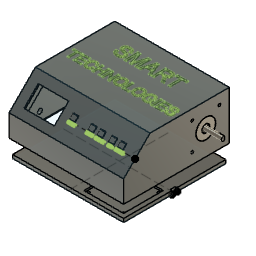
Stepper motor box v1 (Autodesk Fusion 360 design; units mm, degrees)
Autodesk Fusion 360 part; units mm, degrees
(part 1 of 3)
sketch "Sketch1" plane through (0, 0, 0) normal (0, 0, 1) x (1, 0, 0) in component "Stepper Motor"
  line L0 (21.15, -21.15) -> (-21.15, -21.15)
  line L1 (-21.15, -21.15) -> (-21.15, 21.15)
  line L2 (-21.15, 21.15) -> (21.15, 21.15)
  line L3 (21.15, 21.15) -> (21.15, -21.15)
  line L4 (21.15, -21.15) -> (-21.15, 21.15) construction
  line L5 (-21.15, -21.15) -> (21.15, 21.15) construction
  dimension "d2" = 42.3
  dimension "d3" = 42.3
  constraint horizontal L0
  constraint perpendicular L0 L1
  constraint parallel L0 L2
  constraint parallel L1 L3
  constraint coincident L4 origin
  constraint coincident L5 origin
  measures "d2" distance of L1.end L2.end
  measures "d3" distance of L0.end L1.end
extrude "Extrude1" add sketch "Sketch1" along normal blind 23 makes body 1 in component "Stepper Motor"
sketch "Sketch2" plane through (0, 0, 23) normal (0, 0, 1) x (-1, 0, 0) in component "Stepper Motor"
  line L0 (-21.15, -21.15) -> (21.15, -21.15)
  line L1 (21.15, -21.15) -> (21.15, 21.15)
  line L2 (21.15, 21.15) -> (-21.15, 21.15)
  line L3 (-21.15, 21.15) -> (-21.15, -21.15)
  circle A0 centre (0, 0) radius 11
  dimension "d6" = 22
  constraint coincident A0.centre origin
  measures "d6" diameter of A0
extrude "Extrude2" add sketch "Sketch2" along normal blind 2 contours A0 bodies 1 in component "Stepper Motor"
sketch "Sketch3" plane through (0, 0, 25) normal (0, 0, 1) x (-1, 0, 0) in component "Stepper Motor"
  circle A0 centre (0, 0) radius 11
  circle A1 centre (0, 0) radius 4.5
  dimension "d9" = 9
  constraint concentric A0 A1
  measures "d9" diameter of A1
extrude "Extrude3" cut sketch "Sketch3" against normal blind 2 contours A1 bodies 1 in component "Stepper Motor"
sketch "Sketch5" plane through (0, 0, 23) normal (0, 0, 1) x (-1, 0, 0) in component "Stepper Motor"
  circle A0 centre (0, 0) radius 4.5
  circle A1 centre (0, 0) radius 2.5
  dimension "d12" = 5
  constraint coincident A0.centre A1.centre
  measures "d12" diameter of A1
extrude "Extrude4" add sketch "Sketch5" along normal blind 22 contours A1 bodies 1 in component "Stepper Motor"
sketch "Sketch6" plane through (0, 0, 45) normal (0, 0, 1) x (-1, 0, 0) in component "Stepper Motor"
  circle A0 centre (0, 0) radius 2.5
  line L0 (2.1585, -1.2614) -> (-2.1585, -1.2614)
  dimension "d15" = 1.2614
  constraint coincident A0 L0.start
  constraint coincident A0 L0.end
  constraint horizontal L0
  measures "d15" distance of A0.centre L0
extrude "Extrude5" cut sketch "Sketch6" against normal blind 6 contours A0 L0 picked at (-0.5645, -1.4539) bodies 1 in component "Stepper Motor"
sketch "Sketch7" plane through (0, 0, 23) normal (0, 0, 1) x (-1, 0, 0) in component "Stepper Motor"
  circle A0 centre (0, 0) radius 11
  line L0 (-21.15, -21.15) -> (21.15, -21.15)
  line L1 (21.15, -21.15) -> (21.15, 21.15)
  line L2 (21.15, 21.15) -> (-21.15, 21.15)
  line L3 (-21.15, 21.15) -> (-21.15, -21.15)
  circle A1 centre (-15.5, -15.5) radius 1.5
  circle A2 centre (15.5, -15.5) radius 1.5
  circle A3 centre (-15.5, 15.5) radius 1.5
  circle A4 centre (15.5, 15.5) radius 1.5
  dimension "d18" = 3
  dimension "d19" = 3
  dimension "d20" = 3
  dimension "d21" = 3
  dimension "d27" = 5.65
  dimension "d28" = 5.65
  dimension "d29" = 5.65
  dimension "d30" = 5.65
  dimension "d32" = 5.65
  dimension "d33" = 5.65
  dimension "d34" = 5.65
  dimension "d35" = 5.65
  measures "d18" diameter of A1
  measures "d19" diameter of A2
  measures "d20" diameter of A3
  measures "d21" diameter of A4
  measures "d27" distance of L3 A3.centre
  measures "d28" distance of L2 A3.centre
  measures "d29" distance of L1 A2.centre
  measures "d30" distance of L0 A2.centre
  measures "d32" distance of L3 A1.centre
  measures "d33" distance of L0 A1.centre
  measures "d34" distance of L2 A4.centre
  measures "d35" distance of L1 A4.centre
extrude "Extrude6" cut sketch "Sketch7" against normal blind 4.5 contours A1 | A2 | A3 | A4 bodies 1 in component "Stepper Motor"
thread "Thread1" "ISO Metric profile 3.0 M3x0.5 6H" major diameter 3.086 minor diameter 2.529 pitch 0.5 angle 60 resizes the face on face at (14.0019, 15.5748, 20) on bodies 1 in component "Stepper Motor"
thread "Thread2" "ISO Metric profile 3.0 M3x0.5 6H" major diameter 3.086 minor diameter 2.529 pitch 0.5 angle 60 resizes the face on face at (-16.9981, 15.5748, 20) on bodies 1 in component "Stepper Motor"
thread "Thread3" "ISO Metric profile 3.0 M3x0.5 6H" major diameter 3.086 minor diameter 2.529 pitch 0.5 angle 60 resizes the face on face at (-16.9981, -15.4252, 20) on bodies 1 in component "Stepper Motor"
thread "Thread4" "ISO Metric profile 3.0 M3x0.5 6H" major diameter 3.086 minor diameter 2.529 pitch 0.5 angle 60 resizes the face on face at (14.0019, -15.4252, 20) on bodies 1 in component "Stepper Motor"
sketch "Sketch8" plane through (0, 0, 23) normal (0, 0, 1) x (-1, 0, 0) in component "Stepper Motor"
  circle A0 centre (-15.5, -15.5) radius 1.2645
  circle A1 centre (15.5, -15.5) radius 1.2645
  circle A2 centre (-15.5, 15.5) radius 1.2645
  circle A3 centre (15.5, 15.5) radius 1.2645
  circle A4 centre (0, 0) radius 11
  line L0 (-21.15, -21.15) -> (21.15, -21.15)
  line L1 (21.15, -21.15) -> (21.15, 21.15)
  line L2 (21.15, 21.15) -> (-21.15, 21.15)
  line L3 (-21.15, 21.15) -> (-21.15, -21.15)
  line L4 (-20.15, 17.65) -> (-20.15, -17.65)
  line L5 (-17.65, -20.15) -> (17.65, -20.15)
  line L6 (20.15, -17.65) -> (20.15, 17.65)
  line L7 (17.65, 20.15) -> (-17.65, 20.15)
  arc A5 (17.65, -20.15) -> (20.15, -17.65) centre (17.65, -17.65) ccw
  arc A6 (20.15, 17.65) -> (17.65, 20.15) centre (17.65, 17.65) ccw
  arc A7 (-17.65, 20.15) -> (-20.15, 17.65) centre (-17.65, 17.65) ccw
  arc A8 (-20.15, -17.65) -> (-17.65, -20.15) centre (-17.65, -17.65) ccw
  line L8 (17.65, -20.15) -> (17.65, -21.15)
  line L9 (20.15, -17.65) -> (21.15, -17.65)
  line L10 (-20.15, -17.65) -> (-21.15, -17.65)
  line L11 (-17.65, -20.15) -> (-17.65, -21.15)
  line L12 (-17.65, 20.15) -> (-17.65, 21.15)
  line L13 (-20.15, 17.65) -> (-21.15, 17.65)
  line L14 (20.15, 17.65) -> (21.15, 17.65)
  line L15 (17.65, 20.15) -> (17.65, 21.15)
  dimension "d41" = 2.5
  dimension "d42" = 1
  dimension "d43" = 1
  dimension "d44" = 1
  dimension "d45" = 1
  constraint parallel L3 L4
  constraint parallel L0 L5
  constraint parallel L1 L6
  constraint parallel L2 L7
  constraint tangent L6 A5
  constraint tangent L5 A5
  constraint tangent L7 A6
  constraint tangent L6 A6
  constraint equal A5 A6
  constraint tangent L7 A7
  constraint tangent L4 A7
  constraint equal A5 A7
  constraint tangent L4 A8
  constraint tangent L5 A8
  constraint equal A5 A8
  constraint coincident L0 L8.end
  constraint perpendicular L0 L8
  constraint coincident L1 L9.end
  constraint perpendicular L1 L9
  constraint coincident L3 L10.end
  constraint perpendicular L3 L10
  constraint coincident L0 L11.end
  constraint perpendicular L0 L11
  constraint coincident L2 L12.end
  constraint perpendicular L2 L12
  constraint coincident L3 L13.end
  constraint perpendicular L3 L13
  constraint coincident L1 L14.end
  constraint perpendicular L1 L14
  constraint coincident L2 L15.end
  constraint perpendicular L2 L15
  measures "d41" radius of A5
  measures "d42" distance of L1 L6
  measures "d43" distance of L0 L5
  measures "d44" distance of L3 L4
  measures "d45" distance of L2 L7
extrude "Extrude7" cut sketch "Sketch8" against normal up to surface (23 mm away) contours L0 L3 A8 L10 L11 | L0 L1 A5 L8 L9 | L2 L3 A7 L12 L13 | L1 L2 A6 L14 L15 bodies 1 in component "Stepper Motor"
sketch "Sketch1 (2)" plane through (21.15, 0, 0) normal (1, 0, 0) x (0, 1, 0)
  line L0 (17.65, 0) -> (17.65, 23)
  line L1 (17.65, 23) -> (-17.65, 23)
  line L2 (-17.65, 23) -> (-17.65, 0)
  line L3 (-17.65, 0) -> (17.65, 0)
  line L4 (-17.65, 16) -> (17.65, 16)
  line L5 (17.65, 9) -> (-17.65, 9)
  dimension "d48" = 7
  dimension "d49" = 9
  constraint coincident L2 L4.start
  constraint coincident L0 L4.end
  constraint perpendicular L0 L4
  constraint coincident L0 L5.start
  constraint coincident L2 L5.end
  constraint perpendicular L2 L5
  measures "d48" distance of L1 L4
  measures "d49" distance of L3 L5
extrude "Extrude8" cut sketch "Sketch1 (2)" against normal blind 1 contours L0 L2 L4 L5 bodies 1 in component "Stepper Motor"
mirror "Mirror1" about plane through (0, 0, 0) normal (1, 0, 0) of "Extrude8" in component "Stepper Motor"
sketch "Sketch2 (2)" plane through (0, 21.15, 0) normal (0, 1, 0) x (-1, 0, 0)
  line L0 (17.65, 0) -> (17.65, 23)
  line L1 (17.65, 23) -> (-17.65, 23)
  line L2 (-17.65, 23) -> (-17.65, 0)
  line L3 (-17.65, 0) -> (17.65, 0)
  line L4 (-17.65, 16) -> (17.65, 16)
  line L5 (17.65, 9) -> (-17.65, 9)
  dimension "d54" = 7
  dimension "d55" = 9
  constraint coincident L2 L4.start
  constraint coincident L0 L4.end
  constraint perpendicular L0 L4
  constraint coincident L0 L5.start
  constraint coincident L2 L5.end
  constraint perpendicular L2 L5
  measures "d54" distance of L1 L4
  measures "d55" distance of L3 L5
extrude "Extrude9" cut sketch "Sketch2 (2)" against normal blind 1 contours L0 L2 L4 L5 bodies 1 in component "Stepper Motor"
mirror "Mirror2" about plane through (0, 0, 0) normal (0, 1, 0) of "Extrude9" in component "Stepper Motor"
sketch "Sketch4" plane through (0, 0, 0) normal (0, 0, -1) x (1, 0, 0)
  line L0 (-21.15, -17.65) -> (-20.15, -17.65)
  arc A0 (-20.15, -17.65) -> (-17.65, -20.15) centre (-17.65, -17.65) ccw
  line L1 (-17.65, -20.15) -> (-17.65, -21.15)
  line L2 (-17.65, -21.15) -> (17.65, -21.15)
  line L3 (17.65, -21.15) -> (17.65, -20.15)
  arc A1 (17.65, -20.15) -> (20.15, -17.65) centre (17.65, -17.65) ccw
  line L4 (20.15, -17.65) -> (21.15, -17.65)
  line L5 (21.15, -17.65) -> (21.15, 17.65)
  line L6 (21.15, 17.65) -> (20.15, 17.65)
  arc A2 (20.15, 17.65) -> (17.65, 20.15) centre (17.65, 17.65) ccw
  line L7 (17.65, 20.15) -> (17.65, 21.15)
  line L8 (17.65, 21.15) -> (-17.65, 21.15)
  line L9 (-17.65, 21.15) -> (-17.65, 20.15)
  arc A3 (-17.65, 20.15) -> (-20.15, 17.65) centre (-17.65, 17.65) ccw
  line L10 (-20.15, 17.65) -> (-21.15, 17.65)
  line L11 (-21.15, 17.65) -> (-21.15, -17.65)
  circle A4 centre (0, 0) radius 4.5
  circle A5 centre (15.5, 15.5) radius 1.5
  circle A6 centre (-15.5, 15.5) radius 1.5
  circle A7 centre (-15.5, -15.5) radius 1.5
  circle A8 centre (15.5, -15.5) radius 1.5
  dimension "d62" = 9
  dimension "d70" = 3
  dimension "d71" = 3
  dimension "d72" = 3
  dimension "d73" = 3
  dimension "d74" = 5.65
  dimension "d75" = 5.65
  dimension "d76" = 5.65
  dimension "d77" = 5.65
  dimension "d78" = 5.65
  dimension "d79" = 5.65
  dimension "d80" = 5.65
  dimension "d81" = 5.65
  constraint coincident A4.centre origin
  measures "d62" diameter of A4
  measures "d70" diameter of A5
  measures "d71" diameter of A6
  measures "d72" diameter of A7
  measures "d73" diameter of A8
  measures "d74" distance of L11 A6.centre
  measures "d75" distance of L8 A6.centre
  measures "d76" distance of L5 A5.centre
  measures "d77" distance of L8 A5.centre
  measures "d78" distance of L5 A8.centre
  measures "d79" distance of L2 A8.centre
  measures "d80" distance of L2 A7.centre
  measures "d81" distance of L11 A7.centre
extrude "Extrude12" cut sketch "Sketch4" against normal blind 2 contours A4 | A5 | A6 | A7 | A8 bodies 1 in component "Stepper Motor"
sketch "Sketch1 (3)" plane through (0, 0, 0) normal (0, 0, 1) x (1, 0, 0) in component "BOX"
  line L0 (65, -60) -> (-65, -60)
  line L1 (-65, -60) -> (-65, 60)
  line L2 (-65, 60) -> (65, 60)
  line L3 (65, 60) -> (65, -60)
  line L4 (65, -60) -> (-65, 60) construction
  line L5 (-65, -60) -> (65, 60) construction
  dimension "d86" = 130
  dimension "d87" = 120
  constraint horizontal L0
  constraint perpendicular L0 L1
  constraint parallel L0 L2
  constraint parallel L1 L3
  constraint coincident L4 origin
  constraint coincident L5 origin
  measures "d86" distance of L1.end L2.end
  measures "d87" distance of L0.end L1.end
extrude "Extrude1'" add sketch "Sketch1 (3)" along normal blind 55 separate body makes body 2 in component "BOX"
chamfer "Chamfer1" distance 30 angle 45 1 edges at (0, -60, 55) on bodies 2 in component "BOX"
shell "Shell1" thickness 5 removed faces 1 at (-21.6667, 20, 0) on bodies 2 in component "BOX"
sketch "Sketch2 (3)" plane through (0, 0, 0) normal (0, 0, -1) x (1, 0, 0) in component "BOX"
  line L0 (60, 55) -> (60, -55)
  line L1 (60, -55) -> (-60, -55)
  line L2 (-60, -55) -> (-60, 55)
  line L3 (-60, 55) -> (60, 55)
  line L4 (-65, -60) -> (65, -60)
  line L5 (65, -60) -> (65, 60)
  line L6 (65, 60) -> (-65, 60)
  line L7 (-65, 60) -> (-65, -60)
  line L8 (63, 58) -> (63, -58)
  line L9 (63, -58) -> (-63, -58)
  line L10 (-63, -58) -> (-63, 58)
  line L11 (-63, 58) -> (63, 58)
  dimension "d92" = -3
extrude "Extrude2'" cut sketch "Sketch2 (3)" against normal blind 4 contours L8 L9 L10 L11 bodies 2 in component "BOX"
sketch "Sketch7 (2)" plane through (0, -38.9645, 38.9645) normal (0, 0.707107, -0.707107) x (-1, 0, 0) in component "BOX"
  line L0 (-60, 15.6066) -> (-60, -22.6777)
  line L1 (-60, -22.6777) -> (60, -22.6777)
  line L2 (60, -22.6777) -> (60, 15.6066)
  line L3 (60, 15.6066) -> (-60, 15.6066)
  line L4 (19.5, 12.6066) -> (55, 12.6066)
  line L5 (55, 12.6066) -> (55, -21.0934)
  line L6 (55, -21.0934) -> (19.5, -21.0934)
  line L7 (19.5, -21.0934) -> (19.5, 12.6066)
  dimension "d113" = 35.5
  dimension "d114" = 33.7
  dimension "d115" = 3
  dimension "d116" = 5
  constraint horizontal L4
  constraint vertical L5
  constraint horizontal L6
  constraint vertical L7
  measures "d113" distance of L4.start L4.end
  measures "d114" distance of L4.start L6.end
  measures "d115" distance of L3 L4
  measures "d116" distance of L2 L5
extrude "Extrude5'" cut sketch "Sketch7 (2)" against normal blind 3 contours L4 L5 L6 L7 bodies 2 in component "BOX"
sketch "Sketch8 (2)" plane through (0, -41.0858, 41.0858) normal (0, 0.707107, -0.707107) x (-1, 0, 0) in component "BOX"
  line L0 (55, -21.0934) -> (55, 12.6066)
  line L1 (55, 12.6066) -> (19.5, 12.6066)
  line L2 (19.5, 12.6066) -> (19.5, -21.0934)
  line L3 (55, -4.2434) -> (19.5, -4.2434) construction
  line L4 (37.25, 12.6066) -> (34.5083, -10.5297) construction
  line L5 (54.5, -15.7434) -> (20, -15.7434)
  line L6 (20, -15.7434) -> (20, 7.2566)
  line L7 (20, 7.2566) -> (54.5, 7.2566)
  line L8 (54.5, 7.2566) -> (54.5, -15.7434)
  line L9 (54.5, -15.7434) -> (20, 7.2566) construction
  line L10 (20, -15.7434) -> (54.5, 7.2566) construction
  line L11 (19.5, -21.0934) -> (55, -21.0934)
  point P0 (37.25, -4.2434)
  dimension "d119" = 34.5
  dimension "d120" = 23
  constraint midpoint L0 L3.start
  constraint midpoint L2 L3.end
  constraint midpoint L1 L4.start
  constraint horizontal L5
  constraint perpendicular L5 L6
  constraint parallel L5 L7
  constraint parallel L6 L8
  constraint coincident L9 P0
  constraint coincident L10 P0
  constraint midpoint L3 P0
  measures "d119" distance of L6.end L7.end
  measures "d120" distance of L5.end L6.end
extrude "Extrude6'" cut sketch "Sketch8 (2)" against normal up to surface (2 mm away) contours L5 L6 L7 L8 bodies 2 in component "BOX"
sketch "Sketch9" plane through (0, -41.0858, 41.0858) normal (0, 0.707107, -0.707107) x (-1, 0, 0) in component "BOX"
  line L0 (54.5, 7.2566) -> (54.5, -15.7434)
  line L1 (54.5, -15.7434) -> (20, -15.7434)
  line L2 (20, -15.7434) -> (20, 7.2566)
  line L3 (20, 7.2566) -> (54.5, 7.2566)
  line L4 (55, -21.0934) -> (55, 12.6066)
  line L5 (55, 12.6066) -> (19.5, 12.6066)
  line L6 (19.5, 12.6066) -> (19.5, -21.0934)
  circle A0 centre (53.1, 10.7066) radius 1.4
  circle A1 centre (21.4, 10.7066) radius 1.4
  circle A2 centre (21.4, -19.1934) radius 1.4
  circle A3 centre (53.1, -19.1934) radius 1.4
  line L7 (54.5, -21.0934) -> (54.5, 12.6066) construction
  line L8 (20, -21.0934) -> (20, 12.6066) construction
  line L9 (54.5, -20.5934) -> (19.5, -20.5934) construction
  line L10 (20, -37.3934) -> (54.5, -37.3934) construction
  line L11 (20, 12.1066) -> (54.5, 12.1066) construction
  line L12 (19.5, -21.0934) -> (55, -21.0934)
  dimension "d123" = 2.8
  dimension "d124" = 2.8
  dimension "d125" = 2.8
  dimension "d126" = 2.8
  dimension "d130" = 0.5
  dimension "d131" = 0.5
  dimension "d133" = 0.5
  constraint coincident L5 L7.end
  constraint perpendicular L5 L7
  constraint coincident L5 L8.end
  constraint perpendicular L5 L8
  constraint coincident L7 L9.start
  constraint coincident L6 L9.end
  constraint perpendicular L8 L9
  constraint coincident L8 L10.start
  constraint coincident L7 L10.end
  constraint perpendicular L7 L10
  constraint coincident L8 L11.start
  constraint coincident L7 L11.end
  constraint perpendicular L7 L11
  constraint tangent A0 L7
  constraint tangent A0 L11
  constraint tangent A1 L11
  constraint tangent A1 L8
  constraint tangent A2 L8
  constraint tangent A2 L9
  constraint tangent A3 L7
  constraint tangent A3 L9
  measures "d123" diameter of A0
  measures "d124" diameter of A1
  measures "d125" diameter of A2
  measures "d126" diameter of A3
  measures "d130" distance of L6 L8
  measures "d131" distance of L4 L7
  measures "d133" distance of L5 L11
extrude "Extrude7'" add sketch "Sketch9" along normal blind 3.5 contours A0 | A1 | A2 | A3 bodies 2 in component "BOX"
sketch "Sketch11" plane through (60, 0, 0) normal (-1, 0, 0) x (0, -1, 0) in component "BOX"
  line L0 (-55, 4) -> (55, 4)
  line L1 (55, 4) -> (55, 22.9289)
  line L2 (55, 22.9289) -> (27.9289, 50)
  line L3 (27.9289, 50) -> (-55, 50)
  line L4 (-55, 50) -> (-55, 4)
  line L5 (-12.2, 6.7) -> (-54.5, 6.7)
  line L6 (-54.5, 6.7) -> (-54.5, 49)
  line L7 (-54.5, 49) -> (-12.2, 49)
  line L8 (-12.2, 49) -> (-12.2, 6.7)
  line L9 (-12.2, 6.7) -> (-54.5, 49) construction
  line L10 (-54.5, 6.7) -> (-12.2, 49) construction
  circle A0 centre (-48.85, 43.35) radius 1.5
  circle A1 centre (-17.85, 43.35) radius 1.5
  circle A2 centre (-48.85, 12.35) radius 1.5
  circle A3 centre (-17.85, 12.35) radius 1.5
  circle A4 centre (-33.35, 27.85) radius 11.25
  point P0 (-33.35, 27.85)
  dimension "d136" = 42.3
  dimension "d137" = 42.3
  dimension "d138" = 0.5
  dimension "d139" = 1
  dimension "d140" = 3
  dimension "d141" = 3
  dimension "d142" = 3
  dimension "d143" = 3
  dimension "d144" = 5.65
  dimension "d145" = 5.65
  dimension "d146" = 5.65
  dimension "d147" = 5.65
  dimension "d148" = 5.65
  dimension "d149" = 5.65
  dimension "d150" = 5.65
  dimension "d151" = 5.65
  dimension "d152" = 22.5
  constraint horizontal L5
  constraint perpendicular L5 L6
  constraint parallel L5 L7
  constraint parallel L6 L8
  constraint coincident L9 P0
  constraint coincident L10 P0
  constraint coincident P0 A4.centre
  measures "d136" distance of L6.end L7.end
  measures "d137" distance of L5.end L6.end
  measures "d138" distance of L4 L6
  measures "d139" distance of L3 L7
  measures "d140" diameter of A0
  measures "d141" diameter of A1
  measures "d142" diameter of A2
  measures "d143" diameter of A3
  measures "d144" distance of L7 A0.centre
  measures "d145" distance of L6 A0.centre
  measures "d146" distance of L7 A1.centre
  measures "d147" distance of L8 A1.centre
  measures "d148" distance of L6 A2.centre
  measures "d149" distance of L5 A2.centre
  measures "d150" distance of L8 A3.centre
  measures "d151" distance of L5 A3.centre
  measures "d152" diameter of A4
extrude "Extrude8'" cut sketch "Sketch11" against normal up to surface (3 mm away) contours L5 L6 L7 L8 bodies 2 in component "BOX"
extrude "Extrude9'" cut 5 faces at (60, 49.0327, 42.8846) (60, 49.7771, 12.4569) (60, 36.5239, 26.7447) (60, 17.5383, 43.5224) (60, 18.2221, 12.6156) along direction (-1, 0, 0) up to surface end surface through (65, 60, 0) normal (1, 0, 0) offset 0 on bodies 2 bodies 2 in component "BOX"
sketch "Sketch12" plane through (0, -38.9645, 38.9645) normal (0, 0.707107, -0.707107) x (-1, 0, 0) in component "BOX"
  line L0 (55, 12.6066) -> (55, -21.0934)
  line L1 (55, -21.0934) -> (19.5, -21.0934)
  line L2 (19.5, -21.0934) -> (19.5, 12.6066)
  line L3 (19.5, 12.6066) -> (55, 12.6066)
  line L4 (-60, 15.6066) -> (-60, -22.6777)
  line L5 (-60, -22.6777) -> (60, -22.6777)
  line L6 (60, -22.6777) -> (60, 15.6066)
  line L7 (60, 15.6066) -> (-60, 15.6066)
  line L8 (15, -18.3934) -> (-56, -18.3934)
  line L9 (-56, -18.3934) -> (-56, 12.6066)
  line L10 (-56, 12.6066) -> (15, 12.6066)
  line L11 (15, 12.6066) -> (15, -18.3934)
  line L12 (15, -18.3934) -> (-56, 12.6066) construction
  line L13 (-56, -18.3934) -> (15, 12.6066) construction
  line L14 (10.3, -5.3934) -> (4, -5.3934)
  line L15 (4, -5.3934) -> (4, 0.9066)
  line L16 (4, 0.9066) -> (10.3, 0.9066)
  line L17 (10.3, 0.9066) -> (10.3, -5.3934)
  line L18 (10.3, -5.3934) -> (4, 0.9066) construction
  line L19 (4, -5.3934) -> (10.3, 0.9066) construction
  line L20 (-10.5, -5.3934) -> (-16.8, -5.3934)
  line L21 (-16.8, -5.3934) -> (-16.8, 0.9066)
  line L22 (-16.8, 0.9066) -> (-10.5, 0.9066)
  line L23 (-10.5, 0.9066) -> (-10.5, -5.3934)
  line L24 (-10.5, -5.3934) -> (-16.8, 0.9066) construction
  line L25 (-16.8, -5.3934) -> (-10.5, 0.9066) construction
  line L26 (-33.8, -5.3934) -> (-40.1, -5.3934)
  line L27 (-40.1, -5.3934) -> (-40.1, 0.9066)
  line L28 (-40.1, 0.9066) -> (-33.8, 0.9066)
  line L29 (-33.8, 0.9066) -> (-33.8, -5.3934)
  line L30 (-33.8, -5.3934) -> (-40.1, 0.9066) construction
  line L31 (-40.1, -5.3934) -> (-33.8, 0.9066) construction
  line L32 (-20.8, -5.3934) -> (-27.1, -5.3934)
  line L33 (-27.1, -5.3934) -> (-27.1, 0.9066)
  line L34 (-27.1, 0.9066) -> (-20.8, 0.9066)
  line L35 (-20.8, 0.9066) -> (-20.8, -5.3934)
  line L36 (-20.8, -5.3934) -> (-27.1, 0.9066) construction
  line L37 (-27.1, -5.3934) -> (-20.8, 0.9066) construction
  line L38 (-44.1, -5.3934) -> (-50.4, -5.3934)
  line L39 (-50.4, -5.3934) -> (-50.4, 0.9066)
  line L40 (-50.4, 0.9066) -> (-44.1, 0.9066)
  line L41 (-44.1, 0.9066) -> (-44.1, -5.3934)
  line L42 (-44.1, -5.3934) -> (-50.4, 0.9066) construction
  line L43 (-50.4, -5.3934) -> (-44.1, 0.9066) construction
  point P0 (-20.5, -2.8934)
  point P1 (7.15, -2.2434)
  point P2 (-13.65, -2.2434)
  point P3 (-36.95, -2.2434)
  point P4 (-23.95, -2.2434)
  point P5 (-47.25, -2.2434)
  dimension "d163" = 71
  dimension "d164" = 31
  dimension "d165" = 4
  dimension "d166" = 3
  dimension "d167" = 6.3
  dimension "d168" = 6.3
  dimension "d169" = 6.3
  dimension "d170" = 6.3
  dimension "d171" = 6.3
  dimension "d172" = 6.3
  dimension "d173" = 6.3
  dimension "d174" = 6.3
  dimension "d175" = 6.3
  dimension "d176" = 6.3
  dimension "d177" = 18
  dimension "d178" = 18
  dimension "d179" = 18
  dimension "d180" = 18
  dimension "d181" = 18
  dimension "d182" = 11
  dimension "d183" = 14.5
  dimension "d184" = 4
  dimension "d185" = 6.7
  dimension "d186" = 4
  constraint horizontal L8
  constraint perpendicular L8 L9
  constraint parallel L8 L10
  constraint parallel L9 L11
  constraint coincident L12 P0
  constraint coincident L13 P0
  constraint horizontal L14
  constraint perpendicular L14 L15
  constraint parallel L14 L16
  constraint parallel L15 L17
  constraint coincident L18 P1
  constraint coincident L19 P1
  constraint horizontal L20
  constraint perpendicular L20 L21
  constraint parallel L20 L22
  constraint parallel L21 L23
  constraint coincident L24 P2
  constraint coincident L25 P2
  constraint horizontal L26
  constraint perpendicular L26 L27
  constraint parallel L26 L28
  constraint parallel L27 L29
  constraint coincident L30 P3
  constraint coincident L31 P3
  constraint horizontal L32
  constraint perpendicular L32 L33
  constraint parallel L32 L34
  constraint parallel L33 L35
  constraint coincident L36 P4
  constraint coincident L37 P4
  constraint horizontal L38
  constraint perpendicular L38 L39
  constraint parallel L38 L40
  constraint parallel L39 L41
  constraint coincident L42 P5
  constraint coincident L43 P5
  measures "d163" distance of L9.end L10.end
  measures "d164" distance of L8.end L9.end
  measures "d165" distance of L4 L9
  measures "d166" distance of L7 L10
  measures "d167" distance of L15.end L16.end
  measures "d168" distance of L14.end L15.end
  measures "d169" distance of L21.end L22.end
  measures "d170" distance of L20.end L21.end
  measures "d171" distance of L27.end L28.end
  measures "d172" distance of L26.end L27.end
  measures "d173" distance of L33.end L34.end
  measures "d174" distance of L32.end L33.end
  measures "d175" distance of L39.end L40.end
  measures "d176" distance of L38.end L39.end
  measures "d177" distance of L10 L14
  measures "d178" distance of L10 L20
  measures "d179" distance of L10 L32
  measures "d180" distance of L10 L26
  measures "d181" distance of L10 L38
  measures "d182" distance of L11 L15
  measures "d183" distance of L15 L23
  measures "d184" distance of L21 L35
  measures "d185" distance of L29 L33
  measures "d186" distance of L27 L41
extrude "Extrude10" cut sketch "Sketch12" against normal up to surface (2 mm away) contours L8 L9 L10 L11 bodies 2 in component "BOX"
extrude "Extrude11" cut 5 faces at (48.3, -41.2933, 36.6357) (35.9, -39.8083, 38.1206) (25, -41.2933, 36.6357) (12.6, -41.2933, 36.6357) (-8.2, -39.8083, 38.1206) along direction (0, 0.707107, -0.707107) up to surface end surface through (65, -45, 40) normal (0, -0.707107, 0.707107) offset 0 on bodies 2 bodies 2 in component "BOX"
sketch "Sketch13" plane through (-10.3, 0, 0) normal (1, 0, 0) x (0, 1, 0) in component "BOX"
  line L0 (-44.1924, 36.565) -> (-39.7376, 41.0197)
  line L1 (-39.7376, 41.0197) -> (-41.8589, 43.1411)
  line L2 (-41.8589, 43.1411) -> (-46.3137, 38.6863)
  line L3 (-46.3137, 38.6863) -> (-44.1924, 36.565)
  line L4 (-41.5054, 42.7875) -> (-45.9602, 38.3327)
  line L5 (-41.8589, 42.434) -> (-42.2125, 42.7875)
  line L6 (-45.6066, 38.6863) -> (-45.9602, 39.0398)
  dimension "d191" = 0.5
  dimension "d192" = 0.5
  dimension "d193" = 0.5
  constraint coincident L1 L4.start
  constraint coincident L3 L4.end
  constraint perpendicular L3 L4
  constraint coincident L4 L5.start
  constraint coincident L2 L5.end
  constraint perpendicular L2 L5
  constraint coincident L4 L6.start
  constraint coincident L2 L6.end
  constraint perpendicular L2 L6
  measures "d191" distance of L2 L4
  measures "d192" distance of L1 L5
  measures "d193" distance of L3 L6
extrude "Extrude12'" add sketch "Sketch13" along normal blind 6 contours L2 L4 L5 L6 bodies 2 in component "BOX"
sketch "Sketch14" plane through (10.5, 0, 0) normal (1, 0, 0) x (0, 1, 0) in component "BOX"
  line L0 (-44.1924, 36.565) -> (-39.7376, 41.0197)
  line L1 (-39.7376, 41.0197) -> (-41.8589, 43.1411)
  line L2 (-41.8589, 43.1411) -> (-46.3137, 38.6863)
  line L3 (-46.3137, 38.6863) -> (-44.1924, 36.565)
  line L4 (-45.9602, 38.3327) -> (-41.5054, 42.7875)
  line L5 (-41.8589, 42.434) -> (-42.2125, 42.7875)
  line L6 (-45.6066, 38.6863) -> (-45.9602, 39.0398)
  dimension "d196" = 0.5
  dimension "d197" = 0.5
  dimension "d198" = 0.5
  constraint coincident L3 L4.start
  constraint coincident L1 L4.end
  constraint perpendicular L1 L4
  constraint coincident L4 L5.start
  constraint coincident L2 L5.end
  constraint perpendicular L2 L5
  constraint coincident L4 L6.start
  constraint coincident L2 L6.end
  constraint perpendicular L2 L6
  measures "d196" distance of L3 L6
  measures "d197" distance of L1 L5
  measures "d198" distance of L2 L4
extrude "Extrude13" add sketch "Sketch14" along normal blind 6 contours L2 L4 L5 L6 bodies 2 in component "BOX"
sketch "Sketch15" plane through (20.8, 0, 0) normal (1, 0, 0) x (0, 1, 0) in component "BOX"
  line L0 (-44.1924, 36.565) -> (-39.7376, 41.0197)
  line L1 (-39.7376, 41.0197) -> (-41.8589, 43.1411)
  line L2 (-41.8589, 43.1411) -> (-46.3137, 38.6863)
  line L3 (-46.3137, 38.6863) -> (-44.1924, 36.565)
  line L4 (-41.5054, 42.7875) -> (-45.9602, 38.3327)
  line L5 (-45.6066, 38.6863) -> (-45.9602, 39.0398)
  line L6 (-41.8589, 42.434) -> (-42.2125, 42.7875)
  dimension "d201" = 0.5
  dimension "d202" = 0.5
  dimension "d203" = 0.5
  constraint coincident L1 L4.start
  constraint coincident L3 L4.end
  constraint perpendicular L3 L4
  constraint coincident L4 L5.start
  constraint coincident L2 L5.end
  constraint perpendicular L2 L5
  constraint coincident L4 L6.start
  constraint coincident L2 L6.end
  constraint perpendicular L2 L6
  measures "d201" distance of L2 L4
  measures "d202" distance of L3 L5
  measures "d203" distance of L1 L6
extrude "Extrude14" add sketch "Sketch15" along normal blind 6 contours L2 L4 L5 L6 bodies 2 in component "BOX"
sketch "Sketch16" plane through (33.8, 0, 0) normal (1, 0, 0) x (0, 1, 0) in component "BOX"
  line L0 (-44.1924, 36.565) -> (-39.7376, 41.0197)
  line L1 (-39.7376, 41.0197) -> (-41.8589, 43.1411)
  line L2 (-41.8589, 43.1411) -> (-46.3137, 38.6863)
  line L3 (-46.3137, 38.6863) -> (-44.1924, 36.565)
  line L4 (-45.9602, 38.3327) -> (-41.5054, 42.7875)
  line L5 (-41.8589, 42.434) -> (-42.2125, 42.7875)
  line L6 (-45.6066, 38.6863) -> (-45.9602, 39.0398)
  dimension "d206" = 0.5
  dimension "d207" = 0.5
  dimension "d208" = 0.5
  constraint coincident L3 L4.start
  constraint coincident L1 L4.end
  constraint perpendicular L1 L4
  constraint coincident L4 L5.start
  constraint coincident L2 L5.end
  constraint perpendicular L2 L5
  constraint coincident L4 L6.start
  constraint coincident L2 L6.end
  constraint perpendicular L2 L6
  measures "d206" distance of L3 L6
  measures "d207" distance of L1 L5
  measures "d208" distance of L2 L4
extrude "Extrude15" add sketch "Sketch16" along normal blind 6 contours L2 L4 L5 L6 bodies 2 in component "BOX"
sketch "Sketch17" plane through (44.1, 0, 0) normal (1, 0, 0) x (0, 1, 0) in component "BOX"
  line L0 (-44.1924, 36.565) -> (-39.7376, 41.0197)
  line L1 (-39.7376, 41.0197) -> (-41.8589, 43.1411)
  line L2 (-41.8589, 43.1411) -> (-46.3137, 38.6863)
  line L3 (-46.3137, 38.6863) -> (-44.1924, 36.565)
  line L4 (-41.5054, 42.7875) -> (-45.9602, 38.3327)
  line L5 (-41.8589, 42.434) -> (-42.2125, 42.7875)
  line L6 (-45.6066, 38.6863) -> (-45.9602, 39.0398)
  dimension "d211" = 0.5
  dimension "d212" = 0.5
  dimension "d213" = 0.5
  constraint coincident L1 L4.start
  constraint coincident L3 L4.end
  constraint perpendicular L3 L4
  constraint coincident L4 L5.start
  constraint coincident L2 L5.end
  constraint perpendicular L2 L5
  constraint coincident L4 L6.start
  constraint coincident L2 L6.end
  constraint perpendicular L2 L6
  measures "d211" distance of L2 L4
  measures "d212" distance of L3 L6
  measures "d213" distance of L1 L5
extrude "Extrude16" add sketch "Sketch17" along normal blind 6 contours L2 L4 L5 L6 bodies 2 in component "BOX"
sketch "Sketch18" plane through (0, -40.3787, 40.3787) normal (0, 0.707107, -0.707107) x (-1, 0, 0) in component "BOX"
  line L0 (-33.8, 0.9066) -> (-33.8, -5.3934)
  line L1 (-33.8, -5.3934) -> (-40.1, -5.3934)
  line L2 (-40.1, -5.3934) -> (-40.1, 0.9066)
  line L3 (-40.1, 0.9066) -> (-33.8, 0.9066)
  line L4 (10.3, 0.9066) -> (10.3, -5.3934)
  line L5 (10.3, -5.3934) -> (4, -5.3934)
  line L6 (4, -5.3934) -> (4, 0.9066)
  line L7 (4, 0.9066) -> (10.3, 0.9066)
  line L8 (-10.5, 0.9066) -> (-10.5, -5.3934)
  line L9 (-10.5, -5.3934) -> (-16.8, -5.3934)
  line L10 (-16.8, -5.3934) -> (-16.8, 0.9066)
  line L11 (-16.8, 0.9066) -> (-10.5, 0.9066)
  line L12 (-20.8, 0.9066) -> (-20.8, -5.3934)
  line L13 (-20.8, -5.3934) -> (-27.1, -5.3934)
  line L14 (-27.1, -5.3934) -> (-27.1, 0.9066)
  line L15 (-27.1, 0.9066) -> (-20.8, 0.9066)
  line L16 (-44.1, 0.9066) -> (-44.1, -5.3934)
  line L17 (-44.1, -5.3934) -> (-50.4, -5.3934)
  line L18 (-50.4, -5.3934) -> (-50.4, 0.9066)
  line L19 (-50.4, 0.9066) -> (-44.1, 0.9066)
  line L20 (-56, 12.6066) -> (-56, -18.3934)
  line L21 (-56, -18.3934) -> (15, -18.3934)
  line L22 (15, -18.3934) -> (15, 12.6066)
  line L23 (15, 12.6066) -> (-56, 12.6066)
  line L24 (-43.6, -5.8934) -> (-50.9, -5.8934)
  line L25 (-50.9, -5.8934) -> (-50.9, 1.4066)
  line L26 (-50.9, 1.4066) -> (-43.6, 1.4066)
  line L27 (-43.6, 1.4066) -> (-43.6, -5.8934)
  line L28 (-33.3, -5.8934) -> (-40.6, -5.8934)
  line L29 (-40.6, -5.8934) -> (-40.6, 1.4066)
  line L30 (-40.6, 1.4066) -> (-33.3, 1.4066)
  line L31 (-33.3, 1.4066) -> (-33.3, -5.8934)
  line L32 (-20.3, -5.8934) -> (-27.6, -5.8934)
  line L33 (-27.6, -5.8934) -> (-27.6, 1.4066)
  line L34 (-27.6, 1.4066) -> (-20.3, 1.4066)
  line L35 (-20.3, 1.4066) -> (-20.3, -5.8934)
  line L36 (-10, -5.8934) -> (-17.3, -5.8934)
  line L37 (-17.3, -5.8934) -> (-17.3, 1.4066)
  line L38 (-17.3, 1.4066) -> (-10, 1.4066)
  line L39 (-10, 1.4066) -> (-10, -5.8934)
  line L40 (10.8, -5.8934) -> (3.5, -5.8934)
  line L41 (3.5, -5.8934) -> (3.5, 1.4066)
  line L42 (3.5, 1.4066) -> (10.8, 1.4066)
  line L43 (10.8, 1.4066) -> (10.8, -5.8934)
  dimension "d216" = -0.5
  dimension "d217" = -0.5
  dimension "d218" = -0.5
  dimension "d219" = -0.5
  dimension "d220" = -0.5
extrude "Extrude17" cut sketch "Sketch18" against normal up to surface (2 mm away) contours L24 L25 L26 L27 | L28 L29 L30 L31 | L32 L33 L34 L35 | L36 L37 L38 L39 | L40 L41 L42 L43 bodies 2 in component "BOX"
extrude "Extrude19" add 1 faces at (-58.3333, -37.6597, 40.2692) along direction (0, 0.707107, -0.707107) blind 3 on bodies 2 bodies 2 in component "BOX"
chamfer "Chamfer2" distance 2 angle 45 1 edges at (0, -25.8076, 47.8787) on bodies 2 in component "BOX"
sketch "Sketch1 (4)" plane through (0, -15, -0.2995) normal (0, 0, -1) x (1, 0, 0) in component "LID"
  line L0 (-64.0864, -50.5389) -> (-64.0864, 59.4611)
  line L1 (-64.0864, 59.4611) -> (55.9136, 59.4611)
  line L2 (55.9136, 59.4611) -> (55.9136, -50.5389)
  line L3 (55.9136, -50.5389) -> (-64.0864, -50.5389)
  line L4 (-67.0864, 62.4611) -> (-67.0864, -53.5389)
  line L5 (-67.0864, -53.5389) -> (58.9136, -53.5389)
  line L6 (58.9136, -53.5389) -> (58.9136, 62.4611)
  line L7 (58.9136, 62.4611) -> (-67.0864, 62.4611)
extrude "Extrude1''" add sketch "Sketch1 (4)" along normal blind 4 separate body contours L0 L1 L2 L3 | L4 L5 L6 L7 makes body 3 in component "LID"
sketch "Sketch2 (4)" plane through (0, 0, -4.2995) normal (0, 0, -1) x (1, 0, 0) in component "LID"
  line L0 (58.9136, 77.4611) -> (-67.0864, 77.4611)
  line L1 (-67.0864, 77.4611) -> (-67.0864, -38.5389)
  line L2 (-67.0864, -38.5389) -> (58.9136, -38.5389)
  line L3 (58.9136, -38.5389) -> (58.9136, 77.4611)
  line L4 (-67.0864, 19.4611) -> (58.9136, 19.4611) construction
  line L5 (-4.0864, 77.4611) -> (-4.0864, -38.5389) construction
  line L6 (58.9136, 22.4611) -> (56.9136, 22.4611)
  line L7 (56.9136, 22.4611) -> (56.9136, 16.4611)
  line L8 (56.9136, 16.4611) -> (58.9136, 16.4611)
  dimension "d237" = 3
  dimension "d238" = 3
  dimension "d239" = 2
  constraint midpoint L1 L4.start
  constraint midpoint L3 L4.end
  constraint midpoint L0 L5.start
  constraint midpoint L2 L5.end
  constraint coincident L3 L6.start
  constraint perpendicular L3 L6
  constraint perpendicular L6 L7
  constraint coincident L3 L8.end
  constraint perpendicular L3 L8
  measures "d237" distance of L4 L6
  measures "d238" distance of L4 L8
  measures "d239" distance of L3 L7
extrude "Extrude3'" cut sketch "Sketch2 (4)" against normal up to surface (4 mm away) contours L3 L6 L7 L8 bodies 3 in component "LID"
sketch "Sketch3 (2)" plane through (0, 0, -0.2995) normal (0, 0, 1) x (-1, 0, 0) in component "LID"
  line L0 (-58.9136, 22.4611) -> (-56.9136, 22.4611)
  line L1 (-56.9136, 22.4611) -> (-56.9136, 16.4611)
  line L2 (-56.9136, 16.4611) -> (-58.9136, 16.4611)
  line L3 (-58.9136, 16.4611) -> (-58.9136, -38.5389)
  line L4 (-58.9136, -38.5389) -> (67.0864, -38.5389)
  line L5 (67.0864, -38.5389) -> (67.0864, 77.4611)
  line L6 (67.0864, 77.4611) -> (-58.9136, 77.4611)
  line L7 (-58.9136, 77.4611) -> (-58.9136, 22.4611)
  line L8 (-15.9136, -34.5389) -> (65.0864, -34.5389)
  line L9 (65.0864, -34.5389) -> (65.0864, 23.4611)
  line L10 (65.0864, 23.4611) -> (-15.9136, 23.4611)
  line L11 (-15.9136, 23.4611) -> (-15.9136, -34.5389)
  line L12 (-15.9136, -34.5389) -> (65.0864, 23.4611) construction
  line L13 (65.0864, -34.5389) -> (-15.9136, 23.4611) construction
  line L14 (22.5864, 23.4611) -> (27.0864, 23.4611)
  line L15 (27.0864, 23.4611) -> (27.0864, 26.4611)
  line L16 (27.0864, 26.4611) -> (22.5864, 26.4611)
  line L17 (22.5864, 26.4611) -> (22.5864, 23.4611)
  line L18 (26.5864, -34.5389) -> (22.5864, -34.5389)
  line L19 (22.5864, -34.5389) -> (22.5864, -32.5389)
  line L20 (22.5864, -32.5389) -> (26.5864, -32.5389)
  line L21 (26.5864, -32.5389) -> (26.5864, -34.5389)
  point P0 (24.5864, -5.5389)
  dimension "d242" = 81
  dimension "d243" = 58
  dimension "d244" = 2
  dimension "d245" = 4
  dimension "d248" = 4.5
  dimension "d249" = 3
  dimension "d250" = 42.5
  dimension "d251" = 2
  dimension "d252" = 42.5
  dimension "d294" = 4
  constraint horizontal L8
  constraint perpendicular L8 L9
  constraint parallel L8 L10
  constraint parallel L9 L11
  constraint coincident L12 P0
  constraint coincident L13 P0
  constraint horizontal L14
  constraint vertical L15
  constraint horizontal L16
  constraint vertical L17
  constraint coincident L10 L14.start
  constraint coincident L8 L18.start
  constraint horizontal L18
  constraint vertical L19
  constraint horizontal L20
  constraint vertical L21
  measures "d242" distance of L9.end L10.end
  measures "d243" distance of L8.end L9.end
  measures "d244" distance of L5 L9
  measures "d245" distance of L4 L8
  measures "d248" distance of L14.start L14.end
  measures "d249" distance of L14.start L16.end
  measures "d250" distance of L9 L17
  measures "d251" distance of L18.start L20.end
  measures "d252" distance of L9 L19
  measures "d294" distance of L19 L21
extrude "Extrude5''" cut sketch "Sketch3 (2)" against normal up to surface (2 mm away) contours L8 L9 L10 L11 L14 L19 L20 L21 | L10 L14 L15 L16 L17 bodies 3 in component "LID"
sketch "Sketch20" plane through (-60, 0, 0) normal (1, 0, 0) x (0, 1, 0) in component "BOX"
  line L0 (-52.8787, 20.8076) -> (-55, 22.9289)
  line L1 (-55, 22.9289) -> (-55, 4)
  line L2 (-55, 4) -> (55, 4)
  line L3 (55, 4) -> (55, 50)
  line L4 (55, 50) -> (-27.9289, 50)
  line L5 (-27.2218, 49.2929) -> (-27.2218, 46.4645)
  line L6 (-27.2218, 46.4645) -> (-52.8787, 20.8076)
  line L7 (41.5, 6.5) -> (30.5, 6.5)
  line L8 (30.5, 6.5) -> (30.5, 19.5)
  line L9 (30.5, 19.5) -> (41.5, 19.5)
  line L10 (41.5, 19.5) -> (41.5, 6.5)
  line L11 (41.5, 6.5) -> (30.5, 19.5) construction
  line L12 (30.5, 6.5) -> (41.5, 19.5) construction
  line L13 (-27.9289, 50) -> (-27.2218, 49.2929)
  point P0 (36, 13)
  dimension "d255" = 11
  dimension "d256" = 13
  dimension "d257" = 15.5
  dimension "d258" = 24.5
  constraint horizontal L7
  constraint perpendicular L7 L8
  constraint parallel L7 L9
  constraint parallel L8 L10
  constraint coincident L11 P0
  constraint coincident L12 P0
  measures "d255" distance of L8.end L9.end
  measures "d256" distance of L7.end L8.end
  measures "d257" distance of L2 L9
  measures "d258" distance of L3 L8
extrude "Extrude20" cut sketch "Sketch20" against normal up to surface (5 mm away) contours L7 L8 L9 L10 bodies 2 in component "BOX"
sketch "Sketch4 (2)" plane through (0, 0, -0.2995) normal (0, 0, 1) x (-1, 0, 0) in component "LID"
  line L0 (-15.9136, 23.4611) -> (22.5864, 23.4611)
  line L1 (22.5864, 23.4611) -> (22.5864, 26.4611)
  line L2 (22.5864, 26.4611) -> (27.0864, 26.4611)
  line L3 (27.0864, 26.4611) -> (27.0864, 23.4611)
  line L4 (27.0864, 23.4611) -> (65.0864, 23.4611)
  line L5 (65.0864, 23.4611) -> (65.0864, -34.5389)
  line L6 (65.0864, -34.5389) -> (26.5864, -34.5389)
  line L7 (26.5864, -34.5389) -> (26.5864, -32.5389)
  line L8 (26.5864, -32.5389) -> (22.5864, -32.5389)
  line L9 (22.5864, -32.5389) -> (22.5864, -34.5389)
  line L10 (22.5864, -34.5389) -> (-15.9136, -34.5389)
  line L11 (-15.9136, -34.5389) -> (-15.9136, 23.4611)
  line L12 (-58.9136, 22.4611) -> (-56.9136, 22.4611)
  line L13 (-56.9136, 22.4611) -> (-56.9136, 16.4611)
  line L14 (-56.9136, 16.4611) -> (-58.9136, 16.4611)
  line L15 (-58.9136, 16.4611) -> (-58.9136, -38.5389)
  line L16 (-58.9136, -38.5389) -> (67.0864, -38.5389)
  line L17 (67.0864, -38.5389) -> (67.0864, 77.4611)
  line L18 (67.0864, 77.4611) -> (-58.9136, 77.4611)
  line L19 (-58.9136, 77.4611) -> (-58.9136, 22.4611)
  line L20 (-8.9136, 72.4611) -> (-53.9136, 72.4611)
  line L21 (-53.9136, 72.4611) -> (-53.9136, 27.4611)
  line L22 (-53.9136, 27.4611) -> (-8.9136, 27.4611)
  line L23 (-8.9136, 27.4611) -> (-8.9136, 72.4611)
  line L24 (-8.9136, 72.4611) -> (-53.9136, 27.4611) construction
  line L25 (-53.9136, 72.4611) -> (-8.9136, 27.4611) construction
  line L26 (-52.9136, 27.4611) -> (-52.9136, 72.4611) construction
  line L27 (-53.9136, 71.4611) -> (-8.9136, 71.4611) construction
  line L28 (-9.9136, 72.4611) -> (-9.9136, 27.4611) construction
  line L29 (-8.9136, 28.4611) -> (-53.9136, 28.4611) construction
  circle A0 centre (-51.3136, 69.8611) radius 1.4
  circle A1 centre (-11.5136, 69.8611) radius 1.4
  circle A2 centre (-51.3136, 30.0611) radius 1.4
  circle A3 centre (-11.5136, 30.0611) radius 1.4
  point P0 (-31.4136, 49.9611)
  dimension "d261" = 45
  dimension "d262" = 45
  dimension "d263" = 5
  dimension "d264" = 5
  dimension "d265" = 1
  dimension "d266" = 1
  dimension "d267" = 1
  dimension "d268" = 1
  dimension "d269" = 2.8
  dimension "d270" = 2.8
  dimension "d271" = 2.8
  dimension "d272" = 2.8
  dimension "d286" = 1.6
  dimension "d287" = 1.6
  dimension "d288" = 1.6
  dimension "d289" = 1.6
  dimension "d290" = 1.6
  dimension "d291" = 1.6
  dimension "d292" = 1.6
  dimension "d293" = 1.6
  constraint horizontal L20
  constraint perpendicular L20 L21
  constraint parallel L20 L22
  constraint parallel L21 L23
  constraint coincident L24 P0
  constraint coincident L25 P0
  constraint coincident L22 L26.start
  constraint coincident L20 L26.end
  constraint perpendicular L20 L26
  constraint coincident L21 L27.start
  constraint coincident L23 L27.end
  constraint perpendicular L23 L27
  constraint coincident L20 L28.start
  constraint coincident L22 L28.end
  constraint perpendicular L22 L28
  constraint coincident L23 L29.start
  constraint coincident L21 L29.end
  constraint perpendicular L21 L29
  measures "d261" distance of L21.end L22.end
  measures "d262" distance of L20.end L21.end
  measures "d263" distance of L19 L21
  measures "d264" distance of L18 L20
  measures "d265" distance of L22 L29
  measures "d266" distance of L21 L26
  measures "d267" distance of L20 L27
  measures "d268" distance of L23 L28
  measures "d269" diameter of A0
  measures "d270" diameter of A1
  measures "d271" diameter of A2
  measures "d272" diameter of A3
  measures "d286" distance of L29 A3.centre
  measures "d287" distance of L28 A3.centre
  measures "d288" distance of L29 A2.centre
  measures "d289" distance of L26 A2.centre
  measures "d290" distance of L27 A1.centre
  measures "d291" distance of L28 A1.centre
  measures "d292" distance of L26 A0.centre
  measures "d293" distance of L27 A0.centre
extrude "Extrude6''" cut sketch "Sketch4 (2)" against normal up to surface (2 mm away) contours L20 L21 L22 L23 bodies 3 in component "LID"
extrude "Extrude7''" add 4 faces at (50.4893, -30.2939, -0.2995) (11.5416, -30.4343, -0.2995) (11.6174, -69.4062, -0.2995) (50.3112, -69.6587, -0.2995) along direction (0, 0, 1) blind 2 on bodies 3 bodies 3 in component "LID"
sketch "Sketch21" plane through (-60, 0, 0) normal (1, 0, 0) x (0, 1, 0) in component "BOX"
  line L0 (41.5, 19.5) -> (41.5, 6.5)
  line L1 (41.5, 6.5) -> (30.5, 6.5)
  line L2 (30.5, 6.5) -> (30.5, 19.5)
  line L3 (30.5, 19.5) -> (41.5, 19.5)
  line L4 (-52.8787, 20.8076) -> (-55, 22.9289)
  line L5 (-55, 22.9289) -> (-55, 4)
  line L6 (-55, 4) -> (55, 4)
  line L7 (55, 4) -> (55, 50)
  line L8 (55, 50) -> (-27.9289, 50)
  line L9 (-27.2218, 49.2929) -> (-27.2218, 46.4645)
  line L10 (-27.2218, 46.4645) -> (-52.8787, 20.8076)
  circle A0 centre (-30, 14) radius 2.75
  line L11 (-27.9289, 50) -> (-27.2218, 49.2929)
  dimension "d277" = 5.5
  dimension "d278" = 10
  dimension "d279" = 25
  measures "d277" diameter of A0
  measures "d278" distance of L6 A0.centre
  measures "d279" distance of L5 A0.centre
extrude "Extrude21" cut sketch "Sketch21" against normal up to surface (5 mm away) contours A0 bodies 2 in component "BOX"
chamfer "Chamfer3" distance 2 angle 45 1 edges at (0, -52.8787, 20.8076) on bodies 2 in component "BOX"
chamfer "Chamfer4" distance 1 angle 45 1 edges at (0, -27.2218, 46.4645) on bodies 2 in component "BOX"
extrude "Extrude8''" cut 4 faces at (11.5416, -30.4343, 1.7005) (50.4893, -30.2939, 1.7005) (50.3112, -69.6587, 1.7005) (11.6174, -69.4062, 1.7005) along direction (0, 0, 1) up to surface end surface through (0, -15, -4.2995) normal (0, 0, -1) offset 0 on bodies 3 bodies 3 in component "LID"